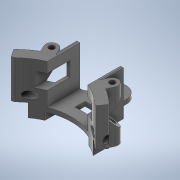
# Autodesk Inventor part: kicker_base_v7
Saved by Autodesk Inventor 2020 (Build 240168000, 168)
## iProperties
Created: 2023-12-16
Part Number: kicker_base_v7
Material: Типовые
Document SubType Name: Modeling
Designer: denis
Density: 1 g/cm^3
Appearance: Гладкая — черная
Author: denis
Autodesk Inventor part; units mm, degrees
(part 1 of 2)
ref_plane "YZ Plane" through (0, 0, 0) normal (1, 0, 0) x (0, 1, 0)
ref_plane "XZ Plane" through (0, 0, 0) normal (0, 1, 0) x (-1, 0, 0)
ref_plane "XY Plane" through (0, 0, 0) normal (0, 0, 1) x (1, 0, 0)
sketch "Эскиз1" plane through (0, 0, 0) normal (0, 1, 0) x (-1, 0, 0)
  line L0 (0, 56.6418) -> (23.7825, 76.5969) construction
  line L1 (44.1942, 76.014) -> (76.014, 44.1942) construction
  line L2 (91.1, 52.2091) -> (52.2091, 91.1) construction
  line L3 (0, 0) -> (74.2462, 74.2462) construction
  arc A0 (92.5543, 49.5852) -> (48.7014, 93.0224) centre (0, 0) ccw construction
  line L4 (52.2091, 91.1) -> (48.6736, 87.5645) construction
  arc A1 (44.1942, 83.085) -> (44.1942, 76.014) centre (47.7297, 79.5495) ccw construction
  line L5 (52.2091, 91.1) -> (48.6736, 87.5645) construction
  line L6 (48.6736, 87.5645) -> (52.2091, 91.1) construction
  spline S0 degree 2 poles (48.6736, 87.5645) (52.2091, 91.1) (48.7014, 93.0224) knots 1 1 1 2 2 2 construction
  line L7 (52.2091, 91.1) -> (48.7014, 93.0224) construction
  line L8 (52.2091, 91.1) -> (48.7014, 93.0224) construction
  arc A2 (48.7014, 93.0224) -> (44.0271, 95.3237) centre (0, 0) ccw construction
  arc A3 (44.0271, 95.3237) -> (43.577, 95.5303) centre (0, 0) ccw construction
  line L9 (42.6652, 95.941) -> (43.577, 95.5303) construction
  line L10 (42.6652, 95.941) -> (43.577, 95.5303) construction
  spline S1 degree 2 poles (42.0492, 94.5734) (42.6652, 95.941) (43.577, 95.5303) knots 1 1 1 2 2 2 construction
  line L11 (42.0492, 94.5734) -> (42.6652, 95.941) construction
  line L12 (42.6652, 95.941) -> (42.0492, 94.5734) construction
  line L13 (0, 0) -> (0, 209.8821) construction
  spline S2 degree 2 poles (-48.6736, 87.5645) (-52.2091, 91.1) (-48.7014, 93.0224) knots 1 1 1 2 2 2 construction
  line L14 (-48.6736, 87.5645) -> (-52.2091, 91.1) construction
  line L15 (-52.2091, 91.1) -> (-48.7014, 93.0224) construction
  arc A4 (-44.1942, 76.014) -> (-44.1942, 83.085) centre (-47.7297, 79.5495) ccw construction
  line L16 (-44.1942, 76.014) -> (-76.014, 44.1942) construction
  arc A5 (-48.7014, 93.0224) -> (-92.5543, 49.5852) centre (0, 0) ccw construction
  arc A6 (-83.085, 44.1942) -> (-76.014, 44.1942) centre (-79.5495, 47.7297) ccw construction
  line L17 (-83.085, 44.1942) -> (-87.3563, 48.4654) construction
  spline S3 degree 2 poles (-48.6736, -87.5645) (-52.2091, -91.1) (-48.7014, -93.0224) knots 1 1 1 2 2 2 construction
  line L18 (-48.6736, -87.5645) -> (-52.2091, -91.1) construction
  line L19 (-52.2091, -91.1) -> (-48.7014, -93.0224) construction
  circle A7 centre (0, 0) radius 35 construction
  line L20 (-46.3155, -73.8927) -> (-73.8927, -46.3155) construction
  arc A8 (-73.8927, -46.3155) -> (-85.2064, -46.3155) centre (-79.5495, -51.9723) ccw construction
  line L21 (-85.2064, -46.3155) -> (-87.5645, -48.6736) construction
  line L22 (-87.5645, -48.6736) -> (-91.1, -52.2091) construction
  spline S4 degree 2 poles (-87.5645, -48.6736) (-91.1, -52.2091) (-92.5543, -49.5852) knots 1 1 1 2 2 2 construction
  line L23 (-91.1, -52.2091) -> (-92.5543, -49.5852) construction
  arc A9 (-92.5543, -49.5852) -> (-48.7014, -93.0224) centre (0, 0) ccw construction
  arc A10 (-92.5543, 49.5852) -> (-92.5543, -49.5852) centre (0, 0) ccw construction
  line L24 (48.6736, -87.5645) -> (46.3155, -85.2064) construction
  arc A11 (-46.3155, -85.2064) -> (-46.3155, -73.8927) centre (-51.9723, -79.5495) ccw construction
  line L25 (-48.6736, -87.5645) -> (-46.3155, -85.2064) construction
  arc A12 (-48.7014, -93.0224) -> (48.7014, -93.0224) centre (0, 0) ccw construction
  arc A13 (46.3155, -73.8927) -> (46.3155, -85.2064) centre (51.9723, -79.5495) ccw construction
  arc A14 (43.577, 95.5303) -> (-43.577, 95.5303) centre (0, 0) ccw construction
  arc A15 (23.7825, 76.5969) -> (0, 67.941) centre (0, 104.941) ccw construction
  line L26 (0, 56.6418) -> (-35.5516, 86.4744) construction
  line L27 (44.0271, 95.3237) -> (44.0271, 127.8162) construction
  ellipse E0 centre (0, 102.7511) end of major axis (44.0271, 102.7511) minor radius 27.5932 (42.0492, 94.5734) -> (35.2734, 86.2384) ccw construction
  line L28 (42.6652, 95.941) -> (-42.6652, 95.941) construction
  ellipse E1 centre (0, 102.7511) end of major axis (44.5159, 105.2445) minor radius 28.887 (35.2734, 86.2384) -> (42.0492, 94.5734) ccw construction
  line L29 (23.7825, 76.5969) -> (35.2734, 86.2384) construction
  arc A16 (0, 67.941) -> (23.7825, 76.5969) centre (0, 104.941) ccw
  arc A17 (-23.7825, 76.5969) -> (0, 67.941) centre (0, 104.941) ccw
  line L30 (-23.7825, 76.5969) -> (-35.2734, 86.2384) construction
  line L31 (-42.6652, 95.941) -> (-42.0492, 94.5734) construction
  arc A18 (-43.577, 95.5303) -> (-48.7014, 93.0224) centre (0, 0) ccw construction
  line L32 (-42.6652, 95.941) -> (-43.577, 95.5303) construction
  spline S5 degree 2 poles (-42.0492, 94.5734) (-42.6652, 95.941) (-43.577, 95.5303) knots 1 1 1 2 2 2 construction
  line L33 (-42.0492, 94.5734) -> (-42.6652, 95.941) construction
  line L34 (-42.6652, 95.941) -> (-43.577, 95.5303) construction
  line L35 (-42.6652, 95.941) -> (-43.577, 95.5303) construction
  spline S6 degree 2 poles (-42.0492, 94.5734) (-42.6652, 95.941) (-43.577, 95.5303) knots 1 1 1 2 2 2 construction
  line L36 (-42.0492, 94.5734) -> (-42.6652, 95.941) construction
  ellipse E2 centre (0, 102.7511) end of major axis (-44.5159, 105.2445) minor radius 28.887 (-42.0492, 94.5734) -> (-35.2734, 86.2384) ccw construction
  line L37 (83.085, 44.1942) -> (87.5645, 48.6736) construction
  arc A19 (76.014, 44.1942) -> (83.085, 44.1942) centre (79.5495, 47.7297) ccw construction
  spline S7 degree 2 poles (48.6736, -87.5645) (52.2091, -91.1) (48.7014, -93.0224) knots 1 1 1 2 2 2 construction
  line L38 (48.6736, -87.5645) -> (52.2091, -91.1) construction
  line L39 (52.2091, -91.1) -> (48.7014, -93.0224) construction
  line L40 (46.3155, -73.8927) -> (73.8927, -46.3155) construction
  arc A20 (85.2064, -46.3155) -> (73.8927, -46.3155) centre (79.5495, -51.9723) ccw construction
  line L41 (85.2064, -46.3155) -> (87.5645, -48.6736) construction
  spline S8 degree 2 poles (87.5645, -48.6736) (91.1, -52.2091) (92.5543, -49.5852) knots 1 1 1 2 2 2 construction
  line L42 (87.5645, -48.6736) -> (91.1, -52.2091) construction
  line L43 (91.1, -52.2091) -> (92.5543, -49.5852) construction
  arc A21 (92.5543, -49.5852) -> (92.5543, 49.5852) centre (0, 0) ccw construction
  arc A22 (48.7014, -93.0224) -> (92.5543, -49.5852) centre (0, 0) ccw construction
  arc A23 (28.5452, 71.4571) -> (-28.5452, 71.4571) centre (0, 104.941) ccw construction
  line L44 (-83.085, 34.2947) -> (-90.6891, 41.8987) construction
  line L45 (-93.5297, 47.6709) -> (-92.5543, 49.5852) construction
  line L46 (-29.1816, 81.127) -> (-76.014, 34.2947) construction
  arc A24 (-83.085, 34.2947) -> (-76.014, 34.2947) centre (-79.5495, 37.8302) ccw construction
  line L47 (-34.1491, 76.1596) -> (-28.5452, 71.4571) construction
  arc A25 (-30.6393, 73.2144) -> (-37.3889, 72.9198) centre (-33.8534, 69.3842) ccw construction
  arc A26 (-90.6891, 41.8987) -> (-87.3563, 48.4654) centre (0, 0) ccw construction
  arc A27 (37.3889, 72.9198) -> (30.6393, 73.2144) centre (33.8534, 69.3842) ccw construction
  line L48 (29.1816, 81.127) -> (76.014, 34.2947) construction
  arc A28 (76.014, 34.2947) -> (83.085, 34.2947) centre (79.5495, 37.8302) ccw construction
  line L49 (83.085, 34.2947) -> (90.6891, 41.8987) construction
  arc A29 (76.014, 44.1942) -> (83.085, 44.1942) centre (79.5495, 47.7297) ccw construction
  line L50 (44.1942, 76.014) -> (76.014, 44.1942) construction
  arc A30 (44.1942, 83.085) -> (44.1942, 76.014) centre (47.7297, 79.5495) ccw construction
  arc A31 (5.5413, 61.2914) -> (28.5452, 71.4571) centre (0, 104.941) ccw
  arc A32 (-28.5452, 71.4571) -> (5.5413, 61.2914) centre (0, 104.941) ccw
  line L51 (34.1491, 76.1596) -> (28.5452, 71.4571) construction
  arc A33 (-87.3563, 48.4654) -> (-90.6891, 41.8987) centre (0, 0) ccw construction
  line L52 (83.085, 44.1942) -> (87.3563, 48.4654) construction
  arc A34 (90.6891, 41.8987) -> (87.3563, 48.4654) centre (0, 0) ccw construction
  line L53 (-44.1942, 83.085) -> (-48.6736, 87.5645) construction
  line L54 (44.0271, 95.3237) -> (43.577, 95.5303) construction
  line L55 (48.6736, 87.5645) -> (44.1942, 83.085) construction
  line L56 (0, 104.941) -> (-23.6028, 54.3247) construction
  circle A35 centre (31.1916, 76.2887) radius 2 construction
  line L57 (29.1816, 81.127) -> (23.7825, 76.5969)
  line L58 (29.1816, 81.127) -> (34.1491, 76.1596)
  line L59 (34.1491, 76.1596) -> (28.5452, 71.4571)
  line L60 (-28.5452, 71.4571) -> (-34.1491, 76.1596)
  line L61 (-23.7825, 76.5969) -> (-29.1816, 81.127)
  line L62 (-29.1816, 81.127) -> (-34.1491, 76.1596)
  arc A36 (-26.6462, 78.9996) -> (-31.2232, 73.7044) centre (-28.9734, 76.3855) ccw
  arc A37 (31.2232, 73.7044) -> (26.6462, 78.9996) centre (28.9734, 76.3855) ccw
  point P0 (60.1041, 60.1041)
  point P1 (40.6586, 79.5495)
  point P2 (79.5495, 40.6586)
  point P3 (0, 105)
  point P4 (-87.5645, 48.6736)
  point P5 (-23.542, 76.3968)
  point P6 (-34.9935, 86.0061)
  point P7 (0, 95.941)
  point P8 (-94.5192, 45.7288)
  point P9 (-13.2817, 58.6489)
  point P10 (-28.5452, 71.4571)
  point P11 (13.2817, 58.6489)
  point P12 (-15.6369, 71.4076)
  point P13 (-26.8032, 79.1314)
  point P14 (-31.2232, 73.7044)
  point P15 (26.8032, 79.1314)
  dimension "d67" = 44.5856
  dimension "d48" = 74
  dimension "d49" = 100
  dimension "d50" = 28
  dimension "d51" = 15
  dimension "d52" = 45
  dimension "d53" = 55
  dimension "d54" = 16.3348
  dimension "d55" = 27.5
  dimension "d56" = 5
  dimension "d57" = 5
  dimension "d58" = 1
  dimension "d59" = 1.5
  dimension "d60" = 1.5
  dimension "d61" = 1
  dimension "d62" = 4
  dimension "d63" = 70
  dimension "d64" = 85
  dimension "d65" = 105
  dimension "d66" = 1.3619
  dimension "d68" = 88
  dimension "d69" = 7
  dimension "d70" = 5
  dimension "d71" = 7
  dimension "d72" = 5
  dimension "d73" = 7
  dimension "d74" = 5
  dimension "d75" = 5.1
  dimension "d78" = 4
  constraints: 91 point on circle, 90 end point, 37 centre point, 28 point on line, 28 symmetric about line, 19 coincident, 17 tangent, 11 collinear, 5 parallel, 4 midpoint, 4 vertical, 3 perpendicular, 1 concentric, 1 equal radius, 68 other
  measures "d48" diameter of A15
  measures "d49" angle of L26 L0
  measures "d50" distance from line of L28 A16.start
  measures "d51" distance of L0.end L29.end
  measures "d52" angle of L13 L3
  measures "d53" distance of point (40.659, 79.55) point (79.55, 40.659)
  measures "d54" distance of L2.start point (79.55, 40.659)
  measures "d55" distance of point (40.659, 79.55) point (60.104, 60.104)
  measures "d56" radius of A1
  measures "d57" distance of L4.start L4.end
  measures "d58" distance of L12.start L10.end
  measures "d59" distance of L12.start L12.end
  measures "d60" distance of L31.start L31.end
  measures "d61" distance of L31.start L35.end
  measures "d62" distance of L4.start L7.end
  measures "d63" diameter of A7
  measures "d64" distance of point (60.104, 60.104) L3.start
  measures "d65" radius of A21
  measures "d66" distance from line of L27 L28.start
  measures "d68" diameter of A23
  measures "d69" distance between parallel lines of L17 L44
  measures "d70" radius of A6
  measures "d71" distance between parallel lines of L46 L16
  measures "d72" radius of A24
  measures "d73" distance between parallel lines of L26 L47
  measures "d74" radius of A25
  measures "d75" radial gap between concentric circles of A10 A26
  measures "d78" diameter of A35
extrude "Выдавливание1" add sketch "Эскиз1" along normal blind 35 contours A16 L57 A37 L59 A31 A32 L60 A36 L61 A17
sketch "Эскиз2" plane through (0, 35, 0) normal (0, 1, 0) x (1, 0, 0)
  arc A0 (92.5543, -49.5852) -> (92.5543, 49.5852) centre (0, 0) ccw construction
  line L0 (90.4123, 37.7305) -> (91.2033, 35.8602)
  arc A1 (91.2033, -35.8602) -> (91.2033, 35.8602) centre (0, 0) ccw construction
  arc A2 (73.8927, 46.3155) -> (85.2064, 46.3155) centre (79.5495, 51.9723) ccw
  arc A3 (90.4123, 37.7305) -> (87.156, 38.3657) centre (88.5702, 36.9514) ccw
  line L1 (87.156, 38.3657) -> (83.085, 34.2947)
  arc A4 (76.014, 34.2947) -> (83.085, 34.2947) centre (79.5495, 37.8302) ccw
  line L2 (-24.842, 61.8893) -> (-23.8313, 59.4808)
  arc A5 (-24.842, 61.8893) -> (-25.4187, 62.8242) centre (-28.1154, 60.5155) ccw
  arc A6 (-48.7014, 93.0224) -> (-92.5543, 49.5852) centre (0, 0) ccw construction
  line L3 (-46.3155, 73.8927) -> (-73.8927, 46.3155)
  line L4 (-76.014, 34.2947) -> (-37.1244, 73.1843)
  line L5 (-91.1, 52.2091) -> (-92.5543, 49.5852) construction
  spline S0 degree 2 poles (-87.5645, 48.6736) (-91.1, 52.2091) (-92.5543, 49.5852) knots 1 1 1 2 2 2
  line L6 (-87.5645, 48.6736) -> (-91.1, 52.2091) construction
  arc A7 (-87.156, 38.3657) -> (-90.4123, 37.7305) centre (-88.5702, 36.9514) ccw
  line L7 (-90.4123, 37.7305) -> (-91.2033, 35.8602)
  line L8 (85.2064, 46.3155) -> (87.5645, 48.6736)
  line L9 (76.014, 34.2947) -> (37.1244, 73.1843)
  line L10 (91.1, 52.2091) -> (87.5645, 48.6736) construction
  line L11 (87.5645, 48.6736) -> (91.1, 52.2091) construction
  line L12 (87.5645, 48.6736) -> (91.1, 52.2091) construction
  spline S1 degree 2 poles (87.5645, 48.6736) (91.1, 52.2091) (92.5543, 49.5852) knots 1 1 1 2 2 2
  line L13 (91.1, 52.2091) -> (92.5543, 49.5852) construction
  line L14 (91.1, 52.2091) -> (92.5543, 49.5852) construction
  line L15 (46.3155, 73.8927) -> (73.8927, 46.3155)
  line L16 (91.1, 52.2091) -> (52.2091, 91.1) construction
  arc A8 (92.5543, 49.5852) -> (48.7014, 93.0224) centre (0, 0) ccw construction
  line L17 (48.6736, 87.5645) -> (46.3155, 85.2064)
  arc A9 (46.3155, 85.2064) -> (46.3155, 73.8927) centre (51.9723, 79.5495) ccw
  arc A10 (25.4187, 62.8242) -> (24.842, 61.8893) centre (28.1154, 60.5155) ccw
  arc A11 (-91.2033, 35.8602) -> (-91.2033, -35.8602) centre (0, 0) ccw construction
  arc A12 (-92.5543, 49.5852) -> (-92.5543, -49.5852) centre (0, 0) ccw construction
  line L18 (0, 0) -> (60.1041, -60.1041) construction
  line L19 (0, 51.8493) -> (0, 56.3493) construction
  line L20 (0.6251, 60.6437) -> (2.0518, 60.1742)
  line L21 (2.672, 59.9702) -> (4.5, 60.5621) construction
  arc A13 (0.6251, 60.6437) -> (-0.6251, 60.6437) centre (0, 58.7439) ccw
  arc A14 (2.0518, 60.1742) -> (3.2931, 60.1713) centre (2.6769, 62.074) ccw
  line L22 (14.5119, 56.4463) -> (0.6161, 51.9466)
  arc A15 (1.5976, 52.1425) -> (2.3373, 52.504) centre (0, 56.3493) ccw construction
  arc A16 (2.672, 59.9702) -> (2.5156, 60.0805) centre (0, 56.3493) ccw construction
  arc A17 (0, 51.8493) -> (0.3604, 51.8638) centre (0, 56.3493) ccw construction
  line L23 (-2.672, 59.9702) -> (-4.5, 60.5621) construction
  arc A18 (-2.5156, 60.0805) -> (-2.672, 59.9702) centre (0, 56.3493) ccw construction
  line L24 (-2.0518, 60.1742) -> (-0.6251, 60.6437)
  arc A19 (-3.2931, 60.1713) -> (-2.0518, 60.1742) centre (-2.6769, 62.074) ccw
  arc A20 (-0.6161, 51.9466) -> (0.6161, 51.9466) centre (0, 53.8493) ccw
  line L25 (-14.5119, 56.4463) -> (-0.6161, 51.9466)
  line L26 (24.842, 61.8893) -> (23.8313, 59.4808)
  line L27 (22.4142, 59.3148) -> (25.4187, 62.8242) construction
  arc A21 (21.5111, 58.7128) -> (22.4142, 59.3148) centre (20.8949, 60.6155) ccw
  arc A22 (21.0049, 57.3328) -> (23.8313, 59.4808) centre (20.5578, 60.8546) ccw
  circle A23 centre (20.5578, 60.8546) radius 1.55
  arc A24 (17.477, 64.7643) -> (18.3802, 65.3664) centre (16.8609, 66.6671) ccw
  line L28 (15.1585, 56.5907) -> (21.0049, 57.3328)
  line L29 (21.5111, 58.7128) -> (14.5119, 56.4463) construction
  arc A25 (15.1585, 56.5907) -> (14.5119, 56.4463) centre (15.6055, 53.069) ccw
  line L30 (0, 0) -> (74.2462, 74.2462) construction
  line L31 (-15.1585, 56.5907) -> (-21.0049, 57.3328)
  arc A26 (-14.5119, 56.4463) -> (-15.1585, 56.5907) centre (-15.6055, 53.069) ccw
  line L32 (25.4187, 62.8242) -> (34.1909, 73.0707)
  line L33 (43.0355, 94.1655) -> (18.3802, 65.3664)
  arc A27 (37.1244, 73.1843) -> (34.1909, 73.0707) centre (35.7102, 71.7701) ccw
  arc A28 (48.7014, 93.0224) -> (45.42, 94.668) centre (0, 0) ccw
  arc A29 (44.0271, 95.3237) -> (43.577, 95.5303) centre (0, 0) ccw construction
  spline S2 degree 2 poles (48.6736, 87.5645) (52.2091, 91.1) (48.7014, 93.0224) knots 1 1 1 2 2 2
  line L34 (48.6736, 87.5645) -> (52.2091, 91.1) construction
  line L35 (52.2091, 91.1) -> (48.7014, 93.0224) construction
  line L36 (52.2091, 91.1) -> (48.6736, 87.5645) construction
  line L37 (52.2091, 91.1) -> (48.6736, 87.5645) construction
  line L38 (52.2091, 91.1) -> (48.7014, 93.0224) construction
  arc A30 (45.42, 94.668) -> (43.0355, 94.1655) centre (44.5548, 92.8648) ccw
  arc A31 (-0.6161, 59.3045) -> (0.6161, 59.3045) centre (0, 61.2072) ccw
  line L39 (17.477, 64.7643) -> (0.6161, 59.3045)
  line L40 (0, 0) -> (0, 95.3237) construction
  line L41 (98, 0) -> (-98, 0) construction
  arc A32 (91.2033, 35.8602) -> (-91.2033, 35.8602) centre (0, 0) ccw construction
  arc A33 (-23.8313, 59.4808) -> (-21.0049, 57.3328) centre (-20.5578, 60.8546) ccw
  line L42 (-20.5578, 60.8546) -> (-24.1768, 56.0927) construction
  line L43 (0, 105) -> (0, 104.941) construction
  arc A34 (-18.3802, 65.3664) -> (-17.477, 64.7643) centre (-16.8609, 66.6671) ccw
  line L44 (-17.477, 64.7643) -> (-0.6161, 59.3045)
  line L45 (0, 104.941) -> (-20.5578, 60.8546) construction
  line L46 (0, 104.941) -> (-23.6028, 54.3247) construction
  line L47 (-20.5578, 60.8546) -> (-22.0043, 58.9513) construction
  circle A35 centre (-20.5578, 60.8546) radius 1.55
  line L48 (-43.0355, 94.1655) -> (-18.3802, 65.3664)
  line L49 (-34.1909, 73.0707) -> (-27.0558, 64.7365) construction
  line L50 (-25.4187, 62.8242) -> (-34.1909, 73.0707)
  arc A36 (-34.1909, 73.0707) -> (-37.1244, 73.1843) centre (-35.7102, 71.7701) ccw
  arc A37 (-22.4142, 59.3148) -> (-21.5111, 58.7128) centre (-20.8949, 60.6155) ccw
  line L51 (-52.2091, 91.1) -> (-48.7014, 93.0224) construction
  spline S3 degree 2 poles (-48.6736, 87.5645) (-52.2091, 91.1) (-48.7014, 93.0224) knots 1 1 1 2 2 2
  line L52 (-48.6736, 87.5645) -> (-52.2091, 91.1) construction
  arc A38 (-46.3155, 73.8927) -> (-46.3155, 85.2064) centre (-51.9723, 79.5495) ccw
  line L53 (-48.6736, 87.5645) -> (-46.3155, 85.2064)
  arc A39 (-45.42, 94.668) -> (-48.7014, 93.0224) centre (0, 0) ccw
  arc A40 (-43.0355, 94.1655) -> (-45.42, 94.668) centre (-44.5548, 92.8648) ccw
  arc A41 (-83.085, 34.2947) -> (-76.014, 34.2947) centre (-79.5495, 37.8302) ccw
  arc A42 (-85.2064, 46.3155) -> (-73.8927, 46.3155) centre (-79.5495, 51.9723) ccw
  line L54 (-85.2064, 46.3155) -> (-87.5645, 48.6736)
  line L55 (-87.156, 38.3657) -> (-83.085, 34.2947)
  circle A43 centre (-79.5495, 37.8302) radius 1.75
  line L56 (-60.1041, 60.1041) -> (-55.1543, 55.1543) construction
  circle A44 centre (-37.8302, 79.5495) radius 1.75
  circle A45 centre (37.8302, 79.5495) radius 1.75
  circle A46 centre (79.5495, 37.8302) radius 1.75
  circle A47 centre (-37.8302, -79.5495) radius 1.75 construction
  arc A48 (-21.0049, -57.3328) -> (-23.8313, -59.4808) centre (-20.5578, -60.8546) ccw construction
  arc A49 (-46.3155, -85.2064) -> (-46.3155, -73.8927) centre (-51.9723, -79.5495) ccw construction
  line L57 (-60.1041, -60.1041) -> (-55.1543, -55.1543) construction
  line L58 (-20.5578, -60.8546) -> (-24.1768, -56.0927) construction
  line L59 (-76.014, -34.2947) -> (-37.1244, -73.1843) construction
  line L60 (-87.5645, -48.6736) -> (-91.1, -52.2091) construction
  spline S4 degree 2 poles (-87.5645, -48.6736) (-91.1, -52.2091) (-92.5543, -49.5852) knots 1 1 1 2 2 2 construction
  line L61 (-91.1, -52.2091) -> (-92.5543, -49.5852) construction
  line L62 (-90.4123, -37.7305) -> (-91.2033, -35.8602) construction
  arc A50 (-90.4123, -37.7305) -> (-87.156, -38.3657) centre (-88.5702, -36.9514) ccw construction
  line L63 (-2.672, -59.9702) -> (-4.5, -60.5621) construction
  arc A51 (0.6161, -59.3045) -> (-0.6161, -59.3045) centre (0, -61.2072) ccw construction
  line L64 (-2.0518, -60.1742) -> (-0.6251, -60.6437) construction
  line L65 (-46.3155, -73.8927) -> (-73.8927, -46.3155) construction
  arc A52 (-92.5543, -49.5852) -> (-48.7014, -93.0224) centre (0, 0) ccw construction
  line L66 (15.1585, -56.5907) -> (21.0049, -57.3328) construction
  line L67 (21.5111, -58.7128) -> (14.5119, -56.4463) construction
  line L68 (0, 0) -> (0, -95.3237) construction
  line L69 (0, 0) -> (74.2462, -74.2462) construction
  line L70 (0.6251, -60.6437) -> (2.0518, -60.1742) construction
  arc A53 (3.2931, -60.1713) -> (2.0518, -60.1742) centre (2.6769, -62.074) ccw construction
  line L71 (2.672, -59.9702) -> (4.5, -60.5621) construction
  line L72 (17.477, -64.7643) -> (0.6161, -59.3045) construction
  line L73 (76.014, -34.2947) -> (37.1244, -73.1843) construction
  arc A54 (83.085, -34.2947) -> (76.014, -34.2947) centre (79.5495, -37.8302) ccw construction
  arc A55 (85.2064, -46.3155) -> (73.8927, -46.3155) centre (79.5495, -51.9723) ccw construction
  arc A56 (-91.2033, -35.8602) -> (91.2033, -35.8602) centre (0, 0) ccw construction
  line L74 (-85.2064, -46.3155) -> (-87.5645, -48.6736) construction
  arc A57 (-73.8927, -46.3155) -> (-85.2064, -46.3155) centre (-79.5495, -51.9723) ccw construction
  circle A58 centre (-79.5495, -37.8302) radius 1.75 construction
  arc A59 (-76.014, -34.2947) -> (-83.085, -34.2947) centre (-79.5495, -37.8302) ccw construction
  line L75 (-87.156, -38.3657) -> (-83.085, -34.2947) construction
  arc A60 (87.156, -38.3657) -> (90.4123, -37.7305) centre (88.5702, -36.9514) ccw construction
  line L76 (90.4123, -37.7305) -> (91.2033, -35.8602) construction
  spline S5 degree 2 poles (87.5645, -48.6736) (91.1, -52.2091) (92.5543, -49.5852) knots 1 1 1 2 2 2 construction
  line L77 (87.5645, -48.6736) -> (91.1, -52.2091) construction
  line L78 (91.1, -52.2091) -> (92.5543, -49.5852) construction
  circle A61 centre (79.5495, -37.8302) radius 1.75 construction
  circle A62 centre (37.8302, -79.5495) radius 1.75 construction
  line L79 (85.2064, -46.3155) -> (87.5645, -48.6736) construction
  line L80 (91.1, -52.2091) -> (87.5645, -48.6736) construction
  line L81 (87.5645, -48.6736) -> (91.1, -52.2091) construction
  line L82 (46.3155, -73.8927) -> (73.8927, -46.3155) construction
  line L83 (91.1, -52.2091) -> (92.5543, -49.5852) construction
  line L84 (91.1, -52.2091) -> (52.2091, -91.1) construction
  arc A63 (48.7014, -93.0224) -> (92.5543, -49.5852) centre (0, 0) ccw construction
  arc A64 (46.3155, -73.8927) -> (46.3155, -85.2064) centre (51.9723, -79.5495) ccw construction
  arc A65 (34.1909, -73.0707) -> (37.1244, -73.1843) centre (35.7102, -71.7701) ccw construction
  line L85 (43.0355, -94.1655) -> (18.3802, -65.3664) construction
  arc A66 (-2.672, -59.9702) -> (-2.5156, -60.0805) centre (0, -56.3493) ccw construction
  line L86 (-15.1585, -56.5907) -> (-21.0049, -57.3328) construction
  arc A67 (-37.1244, -73.1843) -> (-34.1909, -73.0707) centre (-35.7102, -71.7701) ccw construction
  arc A68 (-2.0518, -60.1742) -> (-3.2931, -60.1713) centre (-2.6769, -62.074) ccw construction
  line L87 (-14.5119, -56.4463) -> (-0.6161, -51.9466) construction
  arc A69 (-15.1585, -56.5907) -> (-14.5119, -56.4463) centre (-15.6055, -53.069) ccw construction
  arc A70 (-0.6251, -60.6437) -> (0.6251, -60.6437) centre (0, -58.7439) ccw construction
  arc A71 (2.5156, -60.0805) -> (2.672, -59.9702) centre (0, -56.3493) ccw construction
  line L88 (0, -51.8493) -> (0, -56.3493) construction
  line L89 (14.5119, -56.4463) -> (0.6161, -51.9466) construction
  arc A72 (2.3373, -52.504) -> (1.5976, -52.1425) centre (0, -56.3493) ccw construction
  arc A73 (0.3604, -51.8638) -> (0, -51.8493) centre (0, -56.3493) ccw construction
  arc A74 (0.6161, -51.9466) -> (-0.6161, -51.9466) centre (0, -53.8493) ccw construction
  arc A75 (14.5119, -56.4463) -> (15.1585, -56.5907) centre (15.6055, -53.069) ccw construction
  line L90 (-24.842, -61.8893) -> (-23.8313, -59.4808) construction
  arc A76 (-25.4187, -62.8242) -> (-24.842, -61.8893) centre (-28.1154, -60.5155) ccw construction
  line L91 (-34.1909, -73.0707) -> (-27.0558, -64.7365) construction
  line L92 (-25.4187, -62.8242) -> (-34.1909, -73.0707) construction
  arc A77 (-21.5111, -58.7128) -> (-22.4142, -59.3148) centre (-20.8949, -60.6155) ccw construction
  line L93 (-20.5578, -60.8546) -> (-22.0043, -58.9513) construction
  circle A78 centre (-20.5578, -60.8546) radius 1.55 construction
  line L94 (-48.6736, -87.5645) -> (-46.3155, -85.2064) construction
  spline S6 degree 2 poles (-48.6736, -87.5645) (-52.2091, -91.1) (-48.7014, -93.0224) knots 1 1 1 2 2 2 construction
  line L95 (-48.6736, -87.5645) -> (-52.2091, -91.1) construction
  line L96 (-52.2091, -91.1) -> (-48.7014, -93.0224) construction
  arc A79 (-48.7014, -93.0224) -> (-45.42, -94.668) centre (0, 0) ccw construction
  arc A80 (-45.42, -94.668) -> (-43.0355, -94.1655) centre (-44.5548, -92.8648) ccw construction
  line L97 (-43.0355, -94.1655) -> (-18.3802, -65.3664) construction
  line L98 (25.4187, -62.8242) -> (34.1909, -73.0707) construction
  line L99 (0, -105) -> (0, -104.941) construction
  arc A81 (-17.477, -64.7643) -> (-18.3802, -65.3664) centre (-16.8609, -66.6671) ccw construction
  line L100 (0, -104.941) -> (-20.5578, -60.8546) construction
  line L101 (0, -104.941) -> (-23.6028, -54.3247) construction
  line L102 (-17.477, -64.7643) -> (-0.6161, -59.3045) construction
  arc A82 (24.842, -61.8893) -> (25.4187, -62.8242) centre (28.1154, -60.5155) ccw construction
  arc A83 (22.4142, -59.3148) -> (21.5111, -58.7128) centre (20.8949, -60.6155) ccw construction
  arc A84 (23.8313, -59.4808) -> (21.0049, -57.3328) centre (20.5578, -60.8546) ccw construction
  line L103 (24.842, -61.8893) -> (23.8313, -59.4808) construction
  line L104 (22.4142, -59.3148) -> (25.4187, -62.8242) construction
  arc A85 (18.3802, -65.3664) -> (17.477, -64.7643) centre (16.8609, -66.6671) ccw construction
  circle A86 centre (20.5578, -60.8546) radius 1.55 construction
  line L105 (48.6736, -87.5645) -> (46.3155, -85.2064) construction
  arc A87 (43.0355, -94.1655) -> (45.42, -94.668) centre (44.5548, -92.8648) ccw construction
  spline S7 degree 2 poles (48.6736, -87.5645) (52.2091, -91.1) (48.7014, -93.0224) knots 1 1 1 2 2 2 construction
  line L106 (48.6736, -87.5645) -> (52.2091, -91.1) construction
  line L107 (52.2091, -91.1) -> (48.7014, -93.0224) construction
  line L108 (52.2091, -91.1) -> (48.6736, -87.5645) construction
  line L109 (52.2091, -91.1) -> (48.6736, -87.5645) construction
  arc A88 (45.42, -94.668) -> (48.7014, -93.0224) centre (0, 0) ccw construction
  line L110 (52.2091, -91.1) -> (48.7014, -93.0224) construction
  arc A89 (43.577, -95.5303) -> (44.0271, -95.3237) centre (0, 0) ccw construction
  line L111 (87.156, -38.3657) -> (83.085, -34.2947) construction
  circle A90 centre (-20.5578, -60.8546) radius 1.9
  arc A91 (-18.8674, -64.4798) -> (-16.9326, -59.1641) centre (-20.5578, -60.8546) ccw construction
  line L112 (-24.1831, -62.545) -> (-22.1434, -66.9191)
  arc A92 (28.5452, -71.4571) -> (-28.5452, -71.4571) centre (0, -104.941) ccw construction
  line L113 (-16.9326, -59.1641) -> (-14.893, -63.5381)
  arc A93 (-24.1831, -62.545) -> (-18.8674, -64.4798) centre (-20.5578, -60.8546) ccw construction
  arc A94 (-16.9326, -59.1641) -> (-24.1831, -62.545) centre (-20.5578, -60.8546) ccw
  arc A95 (-14.893, -63.5381) -> (-22.1434, -66.9191) centre (0.0001, -104.9413) ccw
  circle A96 centre (20.5578, -60.8546) radius 1.9
  line L114 (24.1831, -62.545) -> (22.1434, -66.9191)
  line L115 (16.9326, -59.1641) -> (14.893, -63.5381)
  arc A97 (24.1831, -62.545) -> (16.9326, -59.1641) centre (20.5578, -60.8546) ccw
  arc A98 (22.1434, -66.9191) -> (14.893, -63.5381) centre (-0.0001, -104.9413) ccw
  arc A99 (23.7825, -76.5969) -> (-23.7825, -76.5969) centre (0, -104.941) ccw construction
  line L116 (-23.7825, -76.5969) -> (-27.9948, -76.5969) construction
  line L117 (23.7825, -76.5969) -> (27.9948, -76.5969) construction
  point P0 (89.2556, 40.4652)
  point P1 (79.5495, 40.6586)
  point P2 (79.5495, 30.7591)
  point P3 (89.2556, 40.4652)
  point P4 (80.9637, 32.1734)
  point P5 (78.1353, 32.1734)
  point P6 (-23.0382, 57.5909)
  point P7 (-78.1353, 32.1734)
  point P8 (55.1543, 55.1543)
  point P9 (40.6586, 79.5495)
  point P10 (35.5963, 74.7124)
  point P11 (60.1041, 60.1041)
  point P12 (0, 51.7471)
  point P13 (27.0558, 64.7365)
  point P14 (18.0135, 64.938)
  point P15 (0, 59.2072)
  point P16 (0, 59.1049)
  point P17 (0, 66.2072)
  point P18 (-39.283, 89.7822)
  point P19 (-22.7059, 58.0282)
  point P20 (-21.4957, 59.6205)
  point P21 (-18.0135, 64.938)
  point P22 (-44.0271, 95.3237)
  point P23 (-43.577, 95.5303)
  point P24 (-80.9637, 32.1734)
  point P25 (79.5495, 30.7591)
  point P26 (-21.4957, -59.6205)
  point P27 (-22.7059, -58.0282)
  point P28 (-23.0382, -57.5909)
  point P29 (-78.1353, -32.1734)
  point P30 (0, -59.2072)
  point P31 (0, -51.7471)
  point P32 (0, -59.1049)
  point P33 (0, -66.2072)
  point P34 (55.1543, -55.1543)
  point P35 (18.0135, -64.938)
  point P36 (35.5963, -74.7124)
  point P37 (79.5495, -30.7591)
  point P38 (78.1353, -32.1734)
  point P39 (79.5495, -40.6586)
  point P40 (89.2556, -40.4652)
  point P41 (-39.283, -89.7822)
  point P42 (-80.9637, -32.1734)
  point P43 (89.2556, -40.4652)
  point P44 (80.9637, -32.1734)
  point P45 (40.6586, -79.5495)
  point P46 (-44.0271, -95.3237)
  point P47 (-43.577, -95.5303)
  point P48 (27.0558, -64.7365)
  point P49 (-18.0135, -64.938)
  point P50 (79.5495, -30.7591)
  point P51 (0, -67.9475)
  dimension "d140" = 3.1
  dimension "d79" = 16.3348
  dimension "d80" = 27.5
  dimension "d81" = 8
  dimension "d82" = 5
  dimension "d83" = 5
  dimension "d84" = 3
  dimension "d85" = 4
  dimension "d87" = 85
  dimension "d88" = 105
  dimension "d89" = 40
  dimension "d90" = 18.9344
  dimension "d91" = 5.21
  dimension "d92" = 2
  dimension "d93" = 7
  dimension "d94" = 7
  dimension "d95" = 7
  dimension "d96" = 7
  dimension "d97" = 7
  dimension "d98" = 2
  dimension "d99" = 2
  dimension "d100" = 2
  dimension "d101" = 5
  dimension "d102" = 2
  dimension "d119" = 2
  dimension "d131" = 7
  dimension "d133" = 4.5
  dimension "d134" = 2
  dimension "d135" = 5
  dimension "d136" = 5
  dimension "d137" = 0.059
  dimension "d138" = 25
  dimension "d139" = 48.644
  dimension "d141" = 40.567
  dimension "d142" = 1.7087
  dimension "d143" = 120
  dimension "d144" = 3.55
  dimension "d145" = 2
  dimension "d146" = 2.6119
  dimension "d147" = 3.5
  dimension "d148" = 3.8
  dimension "d149" = 8
  constraints: 206 point on circle, 204 end point, 199 symmetric about line, 107 point on line, 96 centre point, 44 tangent, 37 coincident, 12 parallel, 7 equal radius, 4 collinear, 4 perpendicular, 2 horizontal, 2 vertical, 1 midpoint, 92 other
  measures "d79" distance of L10.start point (79.55, 40.659)
  measures "d80" distance of point (40.659, 79.55) point (60.104, 60.104)
  measures "d81" radius of A9
  measures "d82" distance of L16.end L17.start
  measures "d83" distance of L12.start L10.start
  measures "d84" distance of L10.start L13.end
  measures "d85" distance of L16.end L35.end
  measures "d87" distance of point (60.104, 60.104) L30.start
  measures "d88" radius of A0
  measures "d89" distance of A29.start point (18.013, 64.938)
  measures "d90" distance of point (18.013, 64.938) point (0, 59.105)
  measures "d91" distance of A29.start L35.end
  measures "d92" radius of A30
  measures "d93" radial gap between concentric circles of A0 A32
  measures "d94" distance between parallel lines of L15 L9
  measures "d95" distance between parallel lines of L8 L1
  measures "d96" distance between parallel lines of L27 L33
  measures "d97" distance between parallel lines of L39 L29
  measures "d98" radius of A21
  measures "d99" radius of A20
  measures "d100" radius of A27
  measures "d101" distance of point (89.256, 40.465) L0.end
  measures "d102" radius of A3
  measures "d119" radius of A40
  measures "d131" distance of point (0, 66.207) point (0, 59.207)
  measures "d133" distance of L19.start L19.end
  measures "d134" radius of A13
  measures "d135" radius of A4
  measures "d136" radius of A41
  measures "d137" distance of L43.start L43.end
  measures "d138" angle of L40 L46
  measures "d139" distance of L43.end L45.end
  measures "d141" angle of L33 L40
  measures "d142" distance of L47.end point (-23.038, 57.591)
  measures "d143" angle of L2 L31
  measures "d144" radius of A5
  measures "d145" distance of point (-22.706, 58.028) point (-21.496, 59.621)
  measures "d146" distance of L2.start L2.end
  measures "d147" diameter of A43
  measures "d148" diameter of A90
  measures "d149" diameter of A91
extrude "Выдавливание2" add sketch "Эскиз2" against normal blind 35 contours A90 | A94 L113 A95 L112 | A96 | L114 A98 L115 A97
sketch "Эскиз3" plane through (22.1434, 0, 66.9191) normal (0.9063078, 0, 0.4226183) x (0.4226183, 0, -0.9063078)
  line L0 (4.8262, 35) -> (4.8262, 35) construction
  line L1 (4.8262, 35) -> (4.8262, 0) construction
  line L2 (4.8262, 0) -> (4.8262, 0) construction
  line L3 (4.8262, 35) -> (4.8262, 0) construction
  line L4 (2.3262, 35) -> (7.3262, 35) construction
  line L5 (0, 35) -> (0, 0) construction
  line L6 (8.8262, 35) -> (8.8262, 0) construction
  line L7 (8.8262, 35) -> (8.8262, 26.5)
  line L8 (8.8262, 26.5) -> (0, 17.6738)
  line L9 (0, 17.6738) -> (0, 35)
  line L10 (8.8262, 35) -> (4.8262, 35) construction
  line L11 (8.8262, 35) -> (0, 35)
  line L12 (0, 0) -> (8.8262, 0)
  line L13 (-28.7033, 0) -> (-28.7033, 35) construction
  line L14 (8.8262, 0) -> (8.8262, 8.5)
  line L15 (8.8262, 8.5) -> (0, 17.3262)
  line L16 (8.8262, 8.5) -> (8.8262, 26.5)
  line L17 (0, 17.3262) -> (0, 17.6738)
  point P0 (51.2911, 0)
  point P1 (2.3262, 30)
  point P2 (7.3262, 30)
  point P3 (0.5762, 18.25)
  dimension "d156" = 8.5
  dimension "d157" = 45
  dimension "d158" = 8.5
  dimension "d159" = 45
  constraints: 18 end point, 4 point on line, 3 collinear, 1 perpendicular, 1 vertical
  measures "d156" distance of L6.start L7.end
  measures "d157" angle of L6 L8
  measures "d158" distance of L6.end L14.end
  measures "d159" angle of L6 L15
sketch3d "3D эскиз1"
  line L0 (26.8032, 35, 79.1314) -> (23.7825, 35, 76.5969)
  arc A0 (23.7825, 35, 76.5969) -> (-23.7825, 35, 76.5969) centre (0, 35, 104.941) ccw
  line L1 (-23.7825, 35, 76.5969) -> (-26.8032, 35, 79.1314)
sweep "Сдвиг1" cut profiles "Эскиз3" path "3D эскиз1" contours L16 L15 L17 L8
extrude "Выдавливание5" cut sketch "Эскиз2" against normal blind 5 contours A90 | A96
sketch "Эскиз4" plane through (0, 0, 0) normal (0, -1, 0) x (1, 0, 0)
  circle A0 centre (20.5578, 60.8546) radius 1.9 projected
  circle A1 centre (-20.5578, 60.8546) radius 1.9 projected
  point P0 (0, 0)
extrude "Выдавливание6" cut sketch "Эскиз4" against normal blind 15
sketch "Эскиз6" plane through (0, 0, 0) normal (0, -1, 0) x (1, 0, 0)
  circle A0 centre (-20.5578, 60.8546) radius 1.9 construction
  circle A1 centre (20.5578, 60.8546) radius 1.9 construction
  line L0 (31.2232, 73.7044) -> (28.5452, 71.4571) projected
  arc A2 (31.2232, 73.7044) -> (26.8032, 79.1314) centre (28.9734, 76.3855) ccw projected
  line L1 (23.7825, 76.5969) -> (26.8032, 79.1314) projected
  arc A3 (-23.7825, 76.5969) -> (23.7825, 76.5969) centre (0, 104.941) ccw projected
  line L2 (-26.8032, 79.1314) -> (-23.7825, 76.5969) projected
  arc A4 (-26.8032, 79.1314) -> (-31.2232, 73.7044) centre (-28.9734, 76.3855) ccw projected
  line L3 (-28.5452, 71.4571) -> (-31.2232, 73.7044) projected
  arc A5 (-28.5452, 71.4571) -> (-22.1434, 66.9191) centre (0, 104.941) ccw projected
  line L4 (-22.1434, 66.9191) -> (-24.1831, 62.545) construction
  arc A6 (-24.1831, 62.545) -> (-16.9326, 59.1641) centre (-20.5578, 60.8546) ccw construction
  line L5 (-16.9326, 59.1641) -> (-14.893, 63.5381) construction
  arc A7 (-14.893, 63.5381) -> (14.893, 63.5381) centre (0, 104.941) ccw projected
  line L6 (14.893, 63.5381) -> (16.9326, 59.1641) construction
  arc A8 (16.9326, 59.1641) -> (24.1831, 62.545) centre (20.5578, 60.8546) ccw construction
  line L7 (24.1831, 62.545) -> (22.1434, 66.9191) construction
  arc A9 (22.1434, 66.9191) -> (28.5452, 71.4571) centre (0, 104.941) ccw projected
  arc A10 (-23.7825, 76.5969) -> (23.7825, 76.5969) centre (0, 104.941) ccw projected
  line L8 (0, 67.941) -> (0, 60.941) construction
  arc A11 (-14.893, 63.5381) -> (14.893, 63.5381) centre (0, 104.941) ccw construction
  line L9 (-14.893, 63.5381) -> (-14.893, 71.0707)
  line L10 (14.893, 63.5381) -> (14.893, 71.0707)
  arc A12 (-14.893, 71.0707) -> (14.893, 71.0707) centre (0, 104.941) ccw
  line L11 (-22.1434, 66.9191) -> (-22.1434, 75.2987)
  arc A13 (-23.7825, 76.5969) -> (23.7825, 76.5969) centre (0, 104.941) ccw projected
  arc A14 (14.893, 63.5381) -> (22.1434, 66.9191) centre (0, 104.941) ccw projected
  line L12 (22.1434, 66.9191) -> (22.1434, 75.2987)
  point P0 (0, 0)
  constraints: 10 end point, 10 point on circle, 3 vertical, 1 centre point, 1 parallel
extrude "Выдавливание7" cut sketch "Эскиз6" against normal blind 15 contours L0 A9 L12 A3 L1 A2 | A7 L9 A3 L10 | A3 L11 A5 L3 A4 L2
sketch "Эскиз7" plane through (0, 35, 0) normal (0, 1, 0) x (1, 0, 0)
  line L0 (-13, -60.4443) -> (13, -60.4443)
  circle A0 centre (-20.5578, -60.8546) radius 1.9 construction
  circle A1 centre (20.5578, -60.8546) radius 1.9 construction
  line L1 (31.2232, -73.7044) -> (28.5452, -71.4571) construction
  arc A2 (28.5452, -71.4571) -> (22.1434, -66.9191) centre (0, -104.941) ccw construction
  line L2 (22.1434, -66.9191) -> (24.1831, -62.545) construction
  arc A3 (24.1831, -62.545) -> (16.9326, -59.1641) centre (20.5578, -60.8546) ccw construction
  line L3 (16.9326, -59.1641) -> (14.893, -63.5381) construction
  arc A4 (14.893, -63.5381) -> (-14.893, -63.5381) centre (0, -104.941) ccw construction
  line L4 (-14.893, -63.5381) -> (-16.9326, -59.1641) construction
  arc A5 (-16.9326, -59.1641) -> (-24.1831, -62.545) centre (-20.5578, -60.8546) ccw construction
  line L5 (-24.1831, -62.545) -> (-22.1434, -66.9191) construction
  arc A6 (-22.1434, -66.9191) -> (-28.5452, -71.4571) centre (0, -104.941) ccw construction
  line L6 (-28.5452, -71.4571) -> (-31.2232, -73.7044) construction
  arc A7 (-31.2232, -73.7044) -> (-26.8032, -79.1314) centre (-28.9734, -76.3855) ccw construction
  line L7 (-26.8032, -79.1314) -> (-23.7825, -76.5969) construction
  arc A8 (23.7825, -76.5969) -> (-23.7825, -76.5969) centre (0, -104.941) ccw construction
  line L8 (23.7825, -76.5969) -> (26.8032, -79.1314) construction
  arc A9 (26.8032, -79.1314) -> (31.2232, -73.7044) centre (28.9734, -76.3855) ccw construction
  line L9 (0, -67.941) -> (0, -60.941) construction
  line L10 (0, -60.4443) -> (0, -66.4443) construction
  line L11 (-13, -60.4443) -> (-13, -70.3)
  line L12 (13, -60.4443) -> (13, -70.3)
  arc A10 (23.7825, -76.5969) -> (-23.7825, -76.5969) centre (0, -104.941) ccw construction
  line L13 (13, -70.3) -> (-13, -70.3)
  point P0 (0, 0)
  dimension "d168" = 26
  dimension "d169" = 6
  constraints: 12 end point, 4 point on circle, 3 vertical, 1 horizontal, 1 midpoint, 1 perpendicular, 1 symmetric about line
  measures "d168" distance of L0.start L0.end
  measures "d169" distance of L10.start L10.end
extrude "Выдавливание8" cut sketch "Эскиз7" against normal blind 15
ref_plane "РабПлоскость1" through (14.893, 35, 63.5381) normal (0, 0.0000001, 1) x (-1, 0, 0)
sketch "Эскиз9" plane through (14.893, 35, 63.5381) normal (0, 0.0000001, 1) x (-1, 0, 0)
  line L0 (27.893, 0) -> (27.893, 15) construction
  ellipse E0 centre (14.893, 15) end of major axis (-29.107, 15) minor radius 0 (1.893, 15) -> (27.893, 15) ccw construction
  line L1 (1.893, 15) -> (1.893, 0) projected
  ellipse E1 centre (14.893, 0) end of major axis (58.893, 0) minor radius 0 (1.893, 0) -> (0, 0) ccw construction
  line L2 (0, 0) -> (0, 17.3262) construction
  ellipse E2 centre (14.893, 17.3262) end of major axis (58.893, 17.3262) minor radius 0 (0, 17.3262) -> (-7.2505, 17.3262) ccw construction
  line L3 (-7.2505, 17.3262) -> (-7.2505, 0) construction
  ellipse E3 centre (14.893, 0) end of major axis (58.893, 0) minor radius 0 (-7.2505, 0) -> (-13.6522, 0) ccw construction
  line L4 (-13.6522, 17.321) -> (-13.6522, 0) construction
  ellipse E4 centre (14.893, 61.579) end of major axis (54.7049, 101.7567) minor radius 26.3752 (-13.6522, 17.321) -> (-12.8022, 17.3262) ccw construction
  line L5 (-12.8022, 17.3262) -> (-12.8022, 17.6738) construction
  ellipse E5 centre (14.893, -26.579) end of major axis (-24.919, 13.5987) minor radius 26.3752 (-12.8022, 17.6738) -> (-13.6522, 17.679) ccw construction
  line L6 (-13.6522, 20) -> (-13.6522, 17.679) construction
  ellipse E6 centre (14.893, 20) end of major axis (58.893, 20) minor radius 0 (-7.2505, 20) -> (-13.6522, 20) ccw construction
  line L7 (-7.2505, 20) -> (-7.2505, 17.6738) construction
  ellipse E7 centre (14.893, 17.6738) end of major axis (58.893, 17.6738) minor radius 0 (0, 17.6738) -> (-7.2505, 17.6738) ccw construction
  line L8 (0, 17.6738) -> (0, 20) construction
  ellipse E8 centre (14.893, 20) end of major axis (58.893, 20) minor radius 0 (29.7859, 20) -> (0, 20) ccw construction
  line L9 (29.7859, 20) -> (29.7859, 17.6738) construction
  ellipse E9 centre (14.893, 17.6738) end of major axis (58.893, 17.6738) minor radius 0 (37.0364, 17.6738) -> (29.7859, 17.6738) ccw construction
  line L10 (37.0364, 17.6738) -> (37.0364, 20) construction
  ellipse E10 centre (14.893, 20) end of major axis (58.893, 20) minor radius 0 (43.4381, 20) -> (37.0364, 20) ccw construction
  line L11 (43.4381, 20) -> (43.4381, 17.6738) construction
  ellipse E11 centre (14.893, 17.6738) end of major axis (58.893, 17.6738) minor radius 0 (43.7533, 17.6738) -> (43.4381, 17.6738) ccw construction
  line L12 (43.7533, 17.6738) -> (43.7533, 17.3262) construction
  ellipse E12 centre (14.893, 17.3262) end of major axis (58.893, 17.3262) minor radius 0 (43.7533, 17.3262) -> (43.4381, 17.3262) ccw construction
  line L13 (43.4381, 17.3262) -> (43.4381, 0) construction
  ellipse E13 centre (14.893, 0) end of major axis (58.893, 0) minor radius 0 (43.4381, 0) -> (37.0364, 0) ccw construction
  line L14 (37.0364, 0) -> (37.0364, 17.3262) construction
  ellipse E14 centre (14.893, 17.3262) end of major axis (58.893, 17.3262) minor radius 0 (37.0364, 17.3262) -> (29.7859, 17.3262) ccw construction
  line L15 (29.7859, 17.3262) -> (29.7859, 0) construction
  ellipse E15 centre (14.893, 0) end of major axis (58.893, 0) minor radius 0 (29.7859, 0) -> (27.893, 0) ccw construction
  line L16 (1.893, 0) -> (1.893, 15) projected
  line L17 (1.893, 0) -> (-0.107, 0)
  line L18 (-0.107, 0) -> (-0.107, 15)
  line L19 (-0.107, 15) -> (1.893, 15)
  line L20 (1.893, 15) -> (1.893, 9)
  line L21 (14.893, 0) -> (14.893, 17.3262) construction
  line L22 (1.893, 6) -> (3.393, 6) construction
  line L23 (3.393, 6) -> (3.393, 9)
  line L24 (3.393, 9) -> (1.893, 9)
  line L25 (1.893, 9) -> (1.893, 6) construction
  ellipse E16 centre (14.893, 15) end of major axis (-22.107, 15) minor radius 0 (27.893, 15) -> (1.893, 15) ccw construction
  line L26 (1.893, 9) -> (1.893, 6) construction
  line L27 (1.893, 6) -> (1.893, 0)
  line L28 (27.893, 15) -> (27.893, 0)
  line L29 (27.893, 0) -> (27.893, 15)
  line L30 (27.893, 0) -> (29.893, 0)
  line L31 (29.893, 0) -> (29.893, 15)
  line L32 (29.893, 15) -> (27.893, 15)
  line L33 (27.893, 15) -> (27.893, 9)
  line L34 (27.893, 6) -> (26.393, 6) construction
  line L35 (26.393, 6) -> (26.393, 9)
  line L36 (26.393, 9) -> (27.893, 9)
  line L37 (27.893, 9) -> (27.893, 6) construction
  line L38 (27.893, 9) -> (27.893, 6) construction
  line L39 (27.893, 6) -> (27.893, 0)
  line L40 (3.393, 6) -> (1.893, 4.5)
  line L41 (3.393, 6) -> (5.5143, 6) construction
  line L42 (26.393, 6) -> (27.893, 4.5)
  point P0 (14.893, 35)
  point P1 (27.893, 15)
  point P2 (27.893, 9)
  point P3 (1.893, 15)
  point P4 (1.893, 6)
  point P5 (1.893, 9)
  point P6 (27.893, 15)
  point P7 (1.893, 6)
  point P8 (1.893, 9)
  point P9 (27.893, 4.5)
  point P10 (27.893, 6)
  point P11 (1.893, 4.5)
  dimension "d172" = 2
  dimension "d173" = 1.5
  dimension "d174" = 3
  dimension "d175" = 6
  dimension "d178" = 135
  constraints: 52 end point, 11 symmetric about line, 6 parallel, 5 point on line, 2 horizontal, 2 perpendicular, 1 collinear, 1 equal length, 1 vertical, 17 other
  measures "d172" distance of L18.end L19.end
  measures "d173" distance of L24.end L23.end
  measures "d174" distance of L22.end L23.end
  measures "d175" distance from line of point (14.893, 15) L24
  measures "d178" angle of L40 L41
extrude "Выдавливание9" add sketch "Эскиз9" along normal blind 2.5 and the other way blind 15
sketch "Эскиз11" plane through (0, 15, 0) normal (0, -1, 0) x (1, 0, 0)
  arc A0 (-14.893, 63.5381) -> (14.893, 63.5381) centre (0, 104.941) ccw projected
  line L0 (14.893, 71.0707) -> (14.893, 63.5381) projected
  arc A1 (-14.893, 71.0707) -> (14.893, 71.0707) centre (0, 104.941) ccw projected
  line L1 (-14.893, 63.5381) -> (-14.893, 71.0707) projected
  point P0 (0, 0)
extrude "Выдавливание10" add sketch "Эскиз11" along normal blind 10
sketch "Эскиз12" plane through (0, 20, 0) normal (0, 1, 0) x (1, 0, 0)
  arc A0 (13, -70.3) -> (-13, -70.3) centre (0, -104.941) ccw projected
  line L0 (13, -66.0381) -> (13, -70.3) projected
  line L1 (13, -62.9053) -> (13, -66.0381) projected
  arc A1 (13, -62.9053) -> (-13, -62.9053) centre (0, -104.941) ccw projected
  line L2 (-13, -70.3) -> (-13, -62.9053) projected
  point P0 (0, 0)
extrude "Выдавливание11" cut sketch "Эскиз12" against normal blind 7
sketch "Эскиз13" plane through (0, 0, 0) normal (0, 1, 0) x (-1, 0, 0)
  line L0 (0, 0) -> (0, 40) construction
  circle A0 centre (0, 40) radius 1.9
  circle A1 centre (0, 40) radius 4
  dimension "d185" = 40
  dimension "d186" = 3.8
  dimension "d209" = 8
  constraints: 2 centre point, 2 coincident, 2 end point, 1 vertical
  measures "d185" distance of L0.start L0.end
  measures "d186" diameter of A0
  measures "d209" diameter of A1
ref_plane "РабПлоскость2" through (0, 13, 0) normal (0, 1, 0) x (1, 0, 0)
sketch "Эскиз14" plane through (0, 13, 0) normal (0, 1, 0) x (1, 0, 0)
  line L0 (13, -62.9053) -> (13, -70.3) projected
  arc A0 (13, -62.9053) -> (-13, -62.9053) centre (0, -104.941) ccw projected
  line L1 (-13, -70.3) -> (-13, -62.9053) projected
  arc A1 (13, -70.3) -> (-13, -70.3) centre (0, -104.941) ccw projected
  arc A2 (13, -70.3) -> (-13, -70.3) centre (0, -104.941) ccw projected
  line L2 (-8.25, -68.8725) -> (-8.25, -61.7214)
  line L3 (0, -67.941) -> (0, -60.941) construction
  line L4 (8.25, -68.8725) -> (8.25, -61.7214)
  line L5 (-8.25, -61.7214) -> (-8.25, -36.2214)
  line L6 (8.25, -61.7214) -> (8.25, -36.2214)
  line L7 (8.25, -36.2214) -> (-8.25, -36.2214) construction
  line L8 (-8.25, -36.2214) -> (-8.25, -33.9214)
  line L9 (8.25, -36.2214) -> (8.25, -33.9214)
  line L10 (-8.25, -33.9214) -> (8.25, -33.9214)
  line L11 (-8.25, -33.9214) -> (8.25, -33.9214)
  line L12 (8.25, -33.9214) -> (8.25, -30.9214)
  line L13 (8.25, -30.9214) -> (-8.25, -30.9214)
  line L14 (-8.25, -30.9214) -> (-8.25, -33.9214)
  line L15 (-6, -68.4308) -> (-6, -61.352)
  arc A3 (13, -62.9053) -> (-13, -62.9053) centre (0, -104.941) ccw projected
  line L16 (6, -68.4308) -> (6, -61.352)
  line L17 (-6, -54.2214) -> (6, -54.2214)
  line L18 (-6, -61.352) -> (-6, -54.2214)
  line L19 (6, -61.352) -> (6, -54.2214)
  line L20 (-4.5, -68.2157) -> (-4.5, -54.2214)
  line L21 (4.5, -68.2157) -> (4.5, -54.2214)
  point P0 (0, 0)
  dimension "d188" = 16.5
  dimension "d189" = 25.5
  dimension "d190" = 2.3
  dimension "d192" = 3
  dimension "d193" = 7
  dimension "d194" = 18
  dimension "d195" = 1.5
  constraints: 40 end point, 8 symmetric about line, 7 point on circle, 5 vertical, 4 horizontal, 3 parallel, 3 point on line, 2 perpendicular, 1 collinear
  measures "d188" distance between parallel lines of L2 L4
  measures "d189" distance of L2.end L5.end
  measures "d190" distance of L5.end L8.end
  measures "d192" distance of L13.end L8.end
  measures "d193" distance between parallel lines of L1 L15
  measures "d194" distance between parallel lines of L7 L17
  measures "d195" distance between parallel lines of L18 L20
extrude "Выдавливание12" add sketch "Эскиз14" along normal blind 4.5 contours L0 A1 L4 A0 | L4 A1 L16 A0 | A0 L19 L17 L18 L5 L8 L10 L9 L6 | L16 A1 L21 A0 | A0 L21 L17 L19 | L20 A1 L15 A0 | A0 L18 L17 L20 | L15 A1 L2 A0 | L2 A1 L1 A0
extrude "Выдавливание13" add sketch "Эскиз14" along normal blind 6.5 contours L10 L14 L13 L12
ref_plane "РабПлоскость3" through (8.25, 13, 36.2214) normal (0, 0, 1) x (1, 0, 0)
sketch "Эскиз15" plane through (8.25, 13, 36.2214) normal (0, 0, 1) x (1, 0, 0)
  line L0 (0, 4.5) -> (0, 8)
  line L1 (0, 8) -> (-1, 8)
  line L2 (0, 0) -> (0, 4.5) projected
  line L3 (0, 4.5) -> (-3, 4.5)
  line L4 (-3.75, 4.5) -> (4.75, 4.5) projected
  line L5 (-1, 8) -> (-3, 4.5)
  line L6 (-3.75, 0) -> (-12.75, 0) construction
  line L7 (-8.25, 0) -> (-8.25, 4.5) construction
  line L8 (-12.75, 4.5) -> (-3.75, 4.5) construction
  line L9 (-16.5, 4.5) -> (-16.5, 8)
  line L10 (-16.5, 8) -> (-15.5, 8)
  line L11 (-16.5, 4.5) -> (-13.5, 4.5)
  line L12 (-15.5, 8) -> (-13.5, 4.5)
  point P0 (-8.25, -13)
  dimension "d200" = 3.5
  dimension "d201" = 1
  dimension "d202" = 3
  constraints: 18 end point, 4 symmetric about line, 2 midpoint, 1 perpendicular, 1 point on line, 1 vertical
  measures "d200" distance of L0.start L0.end
  measures "d201" distance of L0.end L1.end
  measures "d202" distance of L0.start L3.end